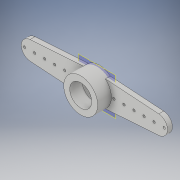
# Autodesk Inventor part: Servo Horn
Saved by Autodesk Inventor 2017 (Build 210142000, 142)
## iProperties
Created: 2016-12-06
Part Number: Servo Horn
Material: Generic
Document SubType Name: Modeling
Designer: PLTW
Density: 1 g/cm^3
Appearance: Default
Author: PLTW
Autodesk Inventor part; units mm, degrees
ref_plane "YZ Plane" through (0, 0, 0) normal (1, 0, 0) x (0, 1, 0)
ref_plane "XZ Plane" through (0, 0, 0) normal (0, 1, 0) x (-1, 0, 0)
ref_plane "XY Plane" through (0, 0, 0) normal (0, 0, 1) x (1, 0, 0)
sketch "Sketch1" plane through (0, 0, 0) normal (0, 0, 1) x (1, 0, 0)
  circle A0 centre (0, 0) radius 3.6957
  dimension "d0" = 7.3914
  constraints: 1 centre point, 1 coincident
  measures "d0" diameter of A0
extrude "Extrusion1" add sketch "Sketch1" along normal blind 4.0386
sketch "Sketch2" plane through (0, 0, 4.0386) normal (0, 0, 1) x (1, 0, 0)
  circle A0 centre (0, 0) radius 3.6957 projected
  circle A1 centre (0, 0) radius 2.4003
  dimension "d3" = 1.2954
  constraints: 1 centre point, 1 coincident
  measures "d3" radial gap between concentric circles of A1 A0
extrude "Extrusion2" cut sketch "Sketch2" against normal blind 2.7432 contours A1
sketch "Sketch3" plane through (0, 0, 0) normal (0, 0, -1) x (-1, 0, 0)
  circle A0 centre (0, 0) radius 3.6957 projected
  circle A1 centre (0, 0) radius 2.1717
  dimension "d6" = 1.524
  constraints: 1 centre point, 1 coincident
  measures "d6" radial gap between concentric circles of A1 A0
extrude "Extrusion3" cut sketch "Sketch3" against normal blind 1.0668 contours A1
sketch "Sketch4" plane through (0, 0, 1.2954) normal (0, 0, 1) x (1, 0, 0)
  circle A0 centre (0, 0) radius 2.4003 projected
  circle A1 centre (0, 0) radius 1.4478
  dimension "d9" = 2.8956
  constraints: 1 centre point, 1 coincident
  measures "d9" diameter of A1
extrude "Extrusion4" cut sketch "Sketch4" against normal through all contours A1
ref_plane "Work Plane1" through (0, 0, 0.5334) normal (0, 0, -1) x (-1, 0, 0)
sketch "Sketch5" plane through (0, 0, 0.5334) normal (0, 0, -1) x (-1, 0, 0)
  circle A0 centre (0, 0) radius 3.6957 projected
  line L0 (-2.3894, 2.8194) -> (-14.0061, 2.032)
  line L1 (-2.3894, -2.8194) -> (-14.0061, -2.032)
  arc A1 (-14.0061, 2.032) -> (-14.0061, -2.032) centre (-13.8684, 0) ccw
  circle A2 centre (0, 0) radius 2.4003 projected
  line L2 (2.3894, 2.8194) -> (14.0061, 2.032)
  arc A3 (14.0061, -2.032) -> (14.0061, 2.032) centre (13.8684, 0) ccw
  line L3 (2.3894, -2.8194) -> (14.0061, -2.032)
  dimension "d12" = 5.6388
  dimension "d13" = 4.064
  dimension "d15" = 13.8684
  dimension "d28" = 360
  constraints: 8 end point, 6 point on circle, 2 centre point, 2 tangent, 1 equal length, 1 horizontal alignment, 17 other
  measures "d12" distance of L1.start L0.start
  measures "d13" distance of L0.end L1.end
  measures "d15" distance of A1.centre point (0, 0)
extrude "Extrusion5" add sketch "Sketch5" along normal mid plane 1.0668 contours A0 L1 A1 L0
sketch "Sketch6" plane through (0, 0, 0) normal (0, 0, -1) x (-1, 0, 0)
  circle A0 centre (0, 0) radius 2.1717 projected
  circle A1 centre (-15.1836, 0) radius 0.2611
  circle A2 centre (-12.9992, 0) radius 0.2611
  circle A3 centre (-10.8148, 0) radius 0.2611
  circle A4 centre (-8.6304, 0) radius 0.2611
  circle A5 centre (-6.446, 0) radius 0.2611
  circle A6 centre (-4.2616, 0) radius 0.2611
  dimension "d18" = 1.8288
  dimension "d19" = 4.0132
  dimension "d20" = 2.1844
  dimension "d21" = 2.1844
  dimension "d22" = 2.1844
  dimension "d23" = 2.1844
  constraints: 6 centre point, 6 horizontal alignment, 5 equal radius
  measures "d20" distance of A4.centre A5.centre
  measures "d21" distance of A4.centre A3.centre
  measures "d22" distance of A2.centre A3.centre
  measures "d23" distance of A1.centre A2.centre
extrude "Extrusion6" cut sketch "Sketch6" against normal through all contours A1 | A2 | A3 | A4 | A5 | A6
pattern_circular "Circular Pattern1" count 2 over 360 about axis through (0, 0, 0) along (0, 0, 1) of "Extrusion5", "Extrusion6"
body "Solid1"
